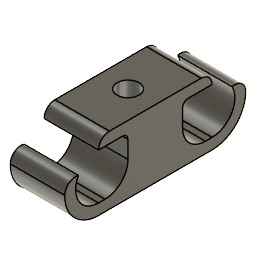
cableClipScrew (Autodesk Fusion 360 archive; units mm, degrees)
design "cableClipScrew" references "variables"
part number: 2026-09-29-17-29-41-598
Autodesk Fusion 360 part; units mm, degrees
derive "ExternalDerived1"
sketch "Sketch1" plane through (0, 0, 0) normal (1, 0, 0) x (0, 1, 0)
  line L0 (-10.4, -3.9) -> (10.4, -3.9)
  arc A0 (10.4, -3.9) -> (10.4, 4.5) centre (10.4, 0.3) ccw
  line L1 (10.4, 4.5) -> (-10.4, 4.5)
  arc A1 (-10.4, 4.5) -> (-10.4, -3.9) centre (-10.4, 0.3) ccw
  line L2 (-10.4, 0.3) -> (10.4, 0.3) construction
  line L3 (-10.4, -5.9) -> (10.4, -5.9)
  arc A2 (10.4, -5.9) -> (10.4, 6.5) centre (10.4, 0.3) ccw
  line L4 (10.4, 6.5) -> (-10.4, 6.5)
  arc A3 (-10.4, 6.5) -> (-10.4, -5.9) centre (-10.4, 0.3) ccw
  line L5 (10.4, 4.5) -> (10.4, 6.5)
  line L6 (-5, 4.5) -> (-5, -3.9)
  line L7 (5, -3.9) -> (5, 4.5)
  line L8 (-10.4, 6.5) -> (-10.4, 4.5)
  line L9 (-14.0859, 2.3134) -> (-15.8412, 3.2722)
  line L10 (-14.0859, 2.3134) -> (-10.4, 0.3)
  line L11 (14.0859, 2.3134) -> (15.8412, 3.2722)
  line L12 (10.4, 0.3) -> (14.0859, 2.3134)
  dimension "d19" = 8.4
  dimension "d23" = 2
  dimension "d62" = 5
  dimension "d63" = 5
  dimension "d66" = 5.4
  dimension "d67" = 5.4
  dimension "d77" = 4.2857
  dimension "d78" = 4.2857
  dimension "d79" = 4.5
  constraint tangent L0 A0
  constraint tangent A0 L1
  constraint parallel L0 L1
  constraint tangent L1 A1
  constraint tangent L0 A1
  constraint horizontal L2
  constraint coincident L1 A0.end
  constraint coincident L4 A2.end
  constraint perpendicular L4 L5
  constraint coincident A2.end L5
  constraint coincident L1 L6.start
  constraint coincident L0 L6.end
  constraint perpendicular L0 L6
  constraint coincident L0 L7.start
  constraint coincident L1 L7.end
  constraint perpendicular L1 L7
  constraint perpendicular L1 L8
  constraint coincident A3 L9.end
  constraint coincident A1 L9.start
  constraint coincident A1.centre L2.start
  constraint collinear L9 L10
  constraint coincident A0 L11.start
  constraint coincident A2 L11.end
  constraint coincident A0.centre L2.end
  constraint collinear L11 L12
  measures "d19" diameter of A0
  measures "d62" distance of origin L6
  measures "d63" distance of origin L7
  measures "d66" distance of A1.centre L6
  measures "d67" distance of A0.centre L7
  measures "d77" distance of L1.end L9.start
  measures "d78" distance of A0.end L11.start
  measures "d79" distance of L1 origin
extrude "Extrude1" add sketch "Sketch1" along normal blind 10 from surface at -5 contours L0 A0 A1 L3 A2 A3 L9 L11 | L0 L1 L6 L7 | L1 L4 L5 L8
sketch "Sketch2" plane through (0, 0, -5.9) normal (0, 0, -1) x (1, 0, 0)
  line L0 (-5, 10.4) -> (-5, -10.4)
  line L1 (-5, -10.4) -> (5, -10.4)
  line L2 (5, -10.4) -> (5, 10.4)
  line L3 (5, 10.4) -> (-5, 10.4)
  circle A0 centre (0, 0) radius 2
  circle A1 centre (0, 0) radius 4
  dimension "d68" = 10.4
  dimension "d69" = 4
  dimension "d74" = 8
  constraint concentric A0 A1
  constraint vertical A0.centre A1.centre
  measures "d68" distance of L3 A0.centre
  measures "d69" diameter of A0
  measures "d74" diameter of A1
extrude "Extrude4" cut sketch "Sketch2" against normal blind 16 contours A0
extrude "Extrude5" cut sketch "Sketch2" against normal blind 8 contours A1
fillet "Fillet7" radius 2 4 edges at (0, 15.8412, 3.2722) (0, 10.4, 6.5) (0, -15.8412, 3.2722) (0, -10.4, 6.5)
fillet "Fillet9" radius 4.2 2 edges at (0, -5, -3.9) (0, 5, -3.9)
fillet "Fillet10" radius 1 2 edges at (0, -5, 4.5) (0, 5, 4.5)
equation "DOWEL_NUMBER_Ref = ceil(( shelf_depth_Ref - dowel_spacing_Ref ) / ( dowel_spacing_Ref + dowel_diameter_Ref ))"
equation "DOWEL_SPACING_Ref = ( shelf_depth_Ref - 2 * edge_spacing_Ref - DOWEL_NUMBER_Ref * dowel_diameter_Ref ) / ( DOWEL_NUMBER_Ref - 1 )"
equation "shelf_height_Ref = 80 mm"
equation "shelf_depth_Ref = 220 mm"
equation "shelf_length_Ref = 1200 mm"
equation "dowel_diameter_Ref = 24 mm"
equation "dowel_spacing_Ref = 18 mm"
equation "edge_spacing_Ref = 10 mm"
equation "support_width_Ref = 25 mm"
equation "support_angle_Ref = 0 deg"
equation "snap_angle_Ref = 90 deg"
equation "mount_edge_spacing_Ref = 25 mm"
equation "hole_diameter_Ref = 8 mm"
equation "hole_length_Ref = 70 mm"
equation "hole_rear_Ref = 20 mm"
equation "mount_thickness_Ref = 7.5 mm"
equation "mount_width_Ref = 200 mm"
equation "mount_depth_Ref = 150 mm"
equation "d19 = cable_diameter * diameter_scaler"
equation "cable_diameter = 6 mm"
equation "num_cables_left = 1"
equation "d23 = thickness"
equation "thickness = 2 mm"
equation "d25 = holder_depth"
equation "clip_thickness = 1.5 mm"
equation "holder_depth = 10 mm"
equation "num_cables_right = 1"
equation "d62 = thickness * 2.5"
equation "d63 = thickness * 2.5"
equation "d66 = num_cables_left * cable_diameter * diameter_scaler - cable_diameter / 2"
equation "d67 = num_cables_right * cable_diameter * diameter_scaler - cable_diameter / 2"
equation "d68 = num_cables_left * cable_diameter * diameter_scaler - cable_diameter / 2 + thickness * 2.5"
equation "d69 = thickness * 2"
equation "d74 = 4 * thickness"
equation "d77 = cable_diameter / diameter_scaler"
equation "d78 = cable_diameter / diameter_scaler"
equation "d79 = 3 * cable_diameter / 4"
equation "d81 = thickness"
equation "d84 = -holder_depth / 2"
equation "d86 = diameter_scaler * cable_diameter / 2"
equation "d88 = thickness / 2"
equation "diameter_scaler = 1.4"
